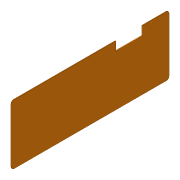
# Autodesk Inventor part: SideFlap
Saved by Autodesk Inventor 2016 (Build 200138000, 138)
## iProperties
Created: 2016-04-01
Part Number: SideFlap
Material: Generic
Document SubType Name: Modeling
Designer: aoben3
Density: 1 g/cm^3
Appearance: Orange
Author: aoben3
Autodesk Inventor part; units mm, degrees
ref_plane "YZ Plane" through (0, 0, 0) normal (1, 0, 0) x (0, 1, 0)
ref_plane "XZ Plane" through (0, 0, 0) normal (0, 1, 0) x (-1, 0, 0)
ref_plane "XY Plane" through (0, 0, 0) normal (0, 0, 1) x (1, 0, 0)
sketch "Sketch1" plane through (0, 0, 0) normal (1, 0, 0) x (0, 1, 0)
  line L0 (-114.3, 300.99) -> (114.3, 300.99)
  line L1 (114.3, 300.99) -> (114.3, -300.99)
  line L2 (114.3, -300.99) -> (-114.3, -300.99)
  line L3 (-114.3, -300.99) -> (-114.3, 300.99)
  line L4 (-114.3, 300.99) -> (114.3, -300.99) construction
  line L5 (114.3, 300.99) -> (-114.3, -300.99) construction
  point P0 (0, 0)
  dimension "d3" = 228.6
  dimension "d4" = 601.98
  constraints: 12 end point, 2 midpoint, 2 parallel, 1 horizontal, 1 perpendicular
  measures "d3" distance of L1.end L2.end
  measures "d4" distance of L2.end L0.start
extrude "Extrusion2" add sketch "Sketch1" along normal blind 2.8575
fillet "Fillet1" radius 10.16 4 edges at (1.4287, -114.3, -300.99) (1.4287, 114.3, -300.99) (1.4287, -114.3, 300.99) (1.4287, 114.3, 300.99)
fillet "Fillet2" radius 0.5715 16 edges at (2.8575, 111.3242, 298.0142) (2.8575, 0, 300.99) (2.8575, -111.3242, 298.0142) (2.8575, -114.3, 0) (2.8575, -111.3242, -298.0142) (2.8575, 0, -300.99) (2.8575, 111.3242, -298.0142) (2.8575, 114.3, 0) (0, 111.3242, -298.0142) (0, 0, -300.99) (0, -111.3242, -298.0142) (0, -114.3, 0) (0, -111.3242, 298.0142) (0, 0, 300.99) (0, 111.3242, 298.0142) (0, 114.3, 0)
sketch "Sketch3" plane through (0, 0, 0) normal (-1, 0, 0) x (0, 0, 1)
  line L0 (300.4185, 104.14) -> (300.4185, -104.14) projected
  line L1 (290.83, -113.7285) -> (-290.83, -113.7285) projected
  line L2 (-290.83, 113.7285) -> (290.83, 113.7285) projected
  line L3 (-300.4185, -104.14) -> (-300.4185, 104.14) projected
  line L4 (290.83, 113.7285) -> (-290.83, 113.7285) projected
  line L5 (-97.2185, 125.0999) -> (-97.2185, 80.4789)
  line L6 (-97.2185, 80.4789) -> (-198.8185, 80.4789)
  line L7 (-198.8185, 80.4789) -> (-198.8185, 125.0999)
  line L8 (-97.2185, 125.0999) -> (-198.8185, 125.0999)
  dimension "d48" = 101.6
  dimension "d49" = 101.6
  dimension "d50" = 0
  dimension "d63" = 11.3714
  dimension "d64" = 33.2496
  constraints: 8 end point, 3 perpendicular, 1 point on line, 1 vertical
  measures "d48" distance between parallel lines of L3 L7
  measures "d49" distance of L5.end L6.end
  measures "d50" distance of L7.end L8.end
  measures "d63" distance between parallel lines of L4 L8
  measures "d64" distance between parallel lines of L4 L6
extrude "Extrusion3" cut sketch "Sketch3" against normal blind 5.08
sketch "Sketch4" plane through (2.8575, 0, 0) normal (1, 0, 0) x (0, 0, -1)
  circle A0 centre (234.3785, 106.1085) radius 2.54
  circle A1 centre (262.3185, 106.1085) radius 2.54
  line L0 (-290.83, 113.7285) -> (290.83, 113.7285) projected
  line L1 (300.4185, 104.14) -> (300.4185, -104.14) projected
  circle A2 centre (-262.89, 106.1085) radius 2.54
  circle A3 centre (-234.95, 106.1085) radius 2.54
  line L2 (-300.99, 104.14) -> (-300.99, -104.14) projected
  point P0 (0, 0)
  point P1 (198.8185, 113.7285)
  dimension "d52" = 5.08
  dimension "d53" = 7.62
  dimension "d54" = 27.94
  dimension "d55" = 38.1
  dimension "d58" = 27.94
  dimension "d60" = 38.1
  constraints: 4 centre point, 3 equal radius, 3 horizontal alignment
  measures "d52" diameter of A0
  measures "d53" distance from line of A0.centre L0
  measures "d54" distance of A1.centre A0.centre
  measures "d55" distance from line of A1.centre L1
  measures "d58" distance of A3.centre A2.centre
  measures "d60" distance from line of A2.centre L2
extrude "Extrusion5" cut sketch "Sketch4" against normal up to next
equation "\"d58\" = d54"
equation "\"d60\" = d55"
equation "\"d61\" = d54"
body "Solid2"
